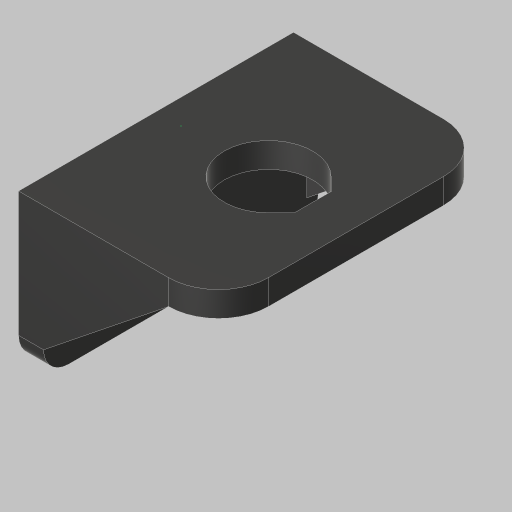
# Autodesk Inventor part: rsl mount
Saved by Autodesk Inventor 2023.5 (Build 275446000, 446)
## iProperties
Created: 2025-02-28
Part Number: rsl mount
Material: ABS Plastic
Document SubType Name: Modeling
Designer: brand
Density: 1.06 g/cm^3
Appearance: Smooth - Black
Author: brand
Autodesk Inventor part; units mm, degrees
ref_plane "YZ Plane" through (0, 0, 0) normal (1, 0, 0) x (0, 1, 0)
ref_plane "XZ Plane" through (0, 0, 0) normal (0, 1, 0) x (-1, 0, 0)
ref_plane "XY Plane" through (0, 0, 0) normal (0, 0, 1) x (1, 0, 0)
sketch "Sketch1" plane through (0, 0, 0) normal (0, 0, 1) x (1, 0, 0)
  line L0 (0, 0) -> (50.8, 0)
  line L1 (50.8, 0) -> (50.8, -6.35)
  line L2 (50.8, -6.35) -> (6.35, -6.35)
  line L3 (6.35, -6.35) -> (6.35, -38.1)
  line L4 (6.35, -38.1) -> (0, -38.1)
  line L5 (0, -38.1) -> (0, 0)
  dimension "d0" = 50.8
  dimension "d1" = 38.1
  dimension "d2" = 6.35
  dimension "d3" = 6.35
  constraints: 12 end point, 5 perpendicular, 1 horizontal
  measures "d0" distance of L0.start L0.end
  measures "d1" distance of L4.end L0.start
  measures "d2" distance of L0.end L1.end
  measures "d3" distance of L3.end L4.end
extrude "Extrusion1" add sketch "Sketch1" along normal mid plane 69.85
sketch "Sketch2" plane through (0, 0, 34.925) normal (0, 1, 0) x (1, 0, 0)
  line L0 (0, 69.85) -> (0, 0) construction
  line L1 (50.8, 0) -> (0, 0) construction
  line L2 (50.8, 69.85) -> (50.8, 0) construction
  line L3 (0, 69.85) -> (50.8, 69.85) construction
  circle A0 centre (28.575, 34.925) radius 11.2522
  line L4 (0, 0) -> (0, 69.85) construction
  line L5 (6.35, 69.85) -> (6.35, 0) construction
  line L6 (6.35, 69.85) -> (6.35, 0) construction
  line L7 (6.35, 69.85) -> (6.35, 0) construction
  line L8 (6.35, 69.85) -> (50.8, 69.85) construction
  line L9 (41.525, 36.525) -> (41.525, 33.325) construction
  line L10 (41.525, 36.525) -> (39.7129, 36.525) construction
  line L11 (41.525, 33.325) -> (39.7129, 33.325) construction
  line L12 (36.5315, 26.9685) -> (44.488, 34.925)
  line L13 (44.488, 34.925) -> (36.5315, 42.8815)
  line L14 (36.5315, 42.8815) -> (39.8272, 42.8815)
  line L15 (39.8272, 42.8815) -> (39.8272, 26.9685)
  line L16 (39.8272, 26.9685) -> (36.5315, 26.9685)
  line L17 (36.5315, 26.9685) -> (36.5315, 42.8815) construction
  point P0 (0, 34.925)
  point P1 (0, 34.925)
  point P2 (28.575, 69.85)
  point P3 (41.525, 34.925)
  point P4 (39.8272, 34.925)
  point P5 (39.8272, 39.5858)
  point P6 (39.8272, 30.2642)
  dimension "d6" = 22.5044
  dimension "d16" = 3.2
  dimension "d17" = 12.95
  constraints: 20 end point, 4 point on circle, 3 horizontal, 3 horizontal alignment, 3 midpoint, 3 perpendicular, 3 tangent, 2 parallel, 1 centre point, 1 vertical, 1 vertical alignment
  measures "d6" diameter of A0
  measures "d16" distance of L9.start L9.end
  measures "d17" distance from line of L9 A0.centre
sketch "Sketch3" plane through (0, -38.1, 34.925) normal (-1, 0, 0) x (0, 0, 1)
  line L0 (0, 0) -> (-69.85, 0) construction
  line L1 (0, 38.1) -> (0, 0) construction
  line L2 (-69.85, 38.1) -> (0, 38.1) construction
  line L3 (-69.85, 0) -> (-69.85, 38.1) construction
  line L4 (-9.525, 25.4) -> (-60.325, 25.4) construction
  line L5 (-60.325, 25.4) -> (-60.325, 12.7) construction
  line L6 (-60.325, 12.7) -> (-9.525, 12.7) construction
  line L7 (-9.525, 12.7) -> (-9.525, 25.4) construction
  line L8 (-9.525, 25.4) -> (-60.325, 12.7) construction
  line L9 (-60.325, 25.4) -> (-9.525, 12.7) construction
  point P0 (-34.925, 38.1)
  point P1 (-34.925, 19.05)
  point P2 (-34.925, 38.1)
  point P3 (0, 19.05)
  point P4 (-34.925, 12.7)
  point P5 (-34.925, 25.4)
  dimension "d7" = 50.8
  dimension "d8" = 12.7
  constraints: 12 end point, 6 midpoint, 4 coincident, 2 parallel, 1 horizontal, 1 horizontal alignment, 1 perpendicular, 1 vertical alignment
  measures "d7" distance of L5.end L6.end
  measures "d8" distance of L4.end L5.end
hole "Hole1" at (0, -12.7, -25.4) at (0, -25.4, -25.4) at (0, -25.4, 25.4) at (0, -12.7, 25.4) direction (1, 0, 0) diameter 5.1054 end through all clearance for "Flat Head Machine Screw (82)" size "#10" standard "Ansi Unified Screw Threads"
extrude "Extrusion2" cut sketch "Sketch2" against normal through all contours A0 | L15 L12 A0 | A0 L13 L15
fillet "Fillet1" [suppressed]
fillet "Fillet2" radius 12.7 2 edges at (50.8, -3.175, -34.925) (50.8, -3.175, 34.925)
fillet "Fillet3" radius 6.35 2 edges at (3.175, -38.1, -34.925) (3.175, -38.1, 34.925)
sketch "Sketch5" plane through (0, 0, -34.925) normal (0, 0, -1) x (-1, 0, 0)
  line L0 (0, -31.75) -> (-6.35, -31.75) construction
  line L1 (0, -31.75) -> (0, 0) construction
  line L2 (0, 0) -> (-38.1, 0) construction
  line L3 (-38.1, -6.35) -> (-38.1, 0) construction
  line L4 (-38.1, -6.35) -> (-6.35, -6.35) construction
  line L5 (-6.35, -6.35) -> (-6.35, -31.75) construction
  line L6 (-38.1, -6.35) -> (-6.35, -31.75)
  line L7 (-6.35, -6.35) -> (-6.35, -31.75)
  line L8 (-6.35, -27.9527) -> (-6.35, -22.8473) construction
  line L9 (-6.35, -6.35) -> (-38.1, -6.35)
  line L10 (-17.3228, -6.35) -> (-17.3228, -6.35) construction
  point P0 (-36.5315, -6.35)
  constraints: 6 end point, 2 collinear
extrude "Extrusion3" add sketch "Sketch5" against normal blind 3
mirror "Mirror1" about plane through (0, 0, 0) normal (0, 0, 1) of "Extrusion3"
fillet "Fillet4" radius 6.35 2 edges at (22.225, -6.35, 31.925) (22.225, -6.35, -31.925)
sketch "Sketch6" plane through (6.35, -38.1, 28.575) normal (1, 0, 0) x (0, 0, -1)
  line L0 (43.4887, 15.24) -> (13.6613, 15.24) construction
  line L1 (13.6613, 15.24) -> (13.6613, 22.86) construction
  line L2 (13.6613, 22.86) -> (43.4887, 22.86) construction
  line L3 (43.4887, 22.86) -> (43.4887, 15.24) construction
  line L4 (50.8, 38.1) -> (6.35, 38.1) construction
  circle A0 centre (3.175, 25.4) radius 2.5527 construction
  circle A1 centre (3.175, 12.7) radius 2.5527 construction
  line L5 (3.175, 25.4) -> (3.175, 12.7) construction
  point P0 (28.575, 38.1)
  point P1 (28.575, 15.24)
  point P2 (28.575, 38.1)
  point P3 (43.4887, 19.05)
  point P4 (3.175, 19.05)
  point P5 (13.6613, 19.05)
  point P6 (28.575, 22.86)
  point P7 (28.575, 38.1)
  dimension "d0" = 50.8
  dimension "d1" = 38.1
  dimension "d2" = 6.35
  dimension "d3" = 6.35
  dimension "d29" = 7.62
  dimension "d30" = 29.8274
  constraints: 7 midpoint, 2 end point, 1 horizontal, 1 horizontal alignment, 1 vertical, 1 vertical alignment, 2 other
  measures "d29" distance of L2.end L0.start
  measures "d30" distance of L0.start L0.end
extrude "Extrusion4" [suppressed]
sketch "Sketch7" plane through (6.35, -38.1, 28.575) normal (1, 0, 0) x (0, 0, -1)
  point P0 (28.575, 38.1)
sketch "Sketch8" plane through (0, 0, -34.925) normal (-1, 0, 0) x (0, 0, 1)
  arc A0 (0, -31.75) -> (6.35, -38.1) centre (6.35, -31.75) ccw construction
  line L0 (0, -31.75) -> (0, 0) construction
  line L1 (0, 0) -> (69.85, 0) construction
  line L2 (69.85, 0) -> (69.85, -31.75) construction
  arc A1 (63.5, -38.1) -> (69.85, -31.75) centre (63.5, -31.75) ccw construction
  line L3 (63.5, -38.1) -> (6.35, -38.1) construction
  circle A2 centre (60.325, -25.4) radius 2.5527 projected
  circle A3 centre (9.525, -12.7) radius 2.5527 projected
  circle A4 centre (9.525, -25.4) radius 2.5527 projected
  circle A5 centre (60.325, -12.7) radius 2.5527 projected
  line L4 (60.325, -25.4) -> (9.525, -25.4) construction
  line L5 (9.525, -25.4) -> (9.525, -12.7) construction
  line L6 (9.525, -12.7) -> (60.325, -12.7) construction
  line L7 (60.325, -12.7) -> (60.325, -25.4) construction
  point P0 (34.925, 0)
  point P1 (34.925, -25.4)
  point P2 (34.925, -12.7)
  constraints: 8 end point, 2 midpoint, 2 parallel, 1 horizontal, 1 perpendicular
hole "Hole2" at (0, -25.4, 0) at (0, -12.7, 0) direction (1, 0, 0) diameter 5.1054 end through all clearance for "Flat Head Machine Screw (82)" size "#10" standard "Ansi Unified Screw Threads"
extrude "Extrusion5" add sketch "Sketch8" against normal up to surface (6.35 mm away)
body "Solid1"
